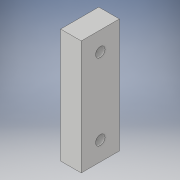
# Autodesk Inventor part: GripperSliderBlock
Saved by Autodesk Inventor 2019 (Build 230136000, 136)
## iProperties
Created: 2019-09-28
Part Number: GripperSliderBlock
Material: Generic
Document SubType Name: Modeling
Designer: james
Density: 1 g/cm^3
Appearance: Default
Mass: 1.5506 g
Surface Area: 10.2449 cm^2
Volume: 1.5506 cm^3
Author: james
Autodesk Inventor part; units mm, degrees
ref_plane "YZ Plane" through (0, 0, 0) normal (1, 0, 0) x (0, 1, 0)
ref_plane "XZ Plane" through (0, 0, 0) normal (0, 1, 0) x (-1, 0, 0)
ref_plane "XY Plane" through (0, 0, 0) normal (0, 0, 1) x (1, 0, 0)
sketch "Sketch1" plane through (0, 0, 0) normal (1, 0, 0) x (0, 1, 0)
  line L0 (12.0622, 21.4347) -> (-26.0378, 21.4347)
  line L1 (-26.0378, 21.4347) -> (-26.0378, 8.7347)
  line L2 (-26.0378, 8.7347) -> (12.0622, 8.7347)
  line L3 (12.0622, 8.7347) -> (12.0622, 21.4347)
  point P0 (0, 0)
  dimension "d0" = 12.7
  dimension "d1" = 38.1
  constraints: 8 end point, 2 parallel, 1 horizontal, 1 perpendicular
  measures "d0" distance of L2.end L0.start
  measures "d1" distance of L0.start L0.end
extrude "Extrusion1" add sketch "Sketch1" along normal blind 6.858
sketch "Sketch2" plane through (6.858, 0, 0) normal (1, 0, 0) x (0, 0, -1)
  line L0 (-8.7347, -26.0378) -> (-8.7347, 12.0622) projected
  line L1 (-8.7347, 12.0622) -> (-21.4347, 12.0622) projected
  point P0 (0, 0)
  point P1 (-15.0847, 5.7122)
  point P2 (-15.0847, -19.6878)
  dimension "d4" = 6.35
  dimension "d5" = 6.35
  dimension "d6" = 31.75
  dimension "d7" = 6.35
  measures "d4" distance from line of L0 point (-15.085, 5.712)
  measures "d5" distance from line of L0 point (-15.085, -19.688)
  measures "d6" distance from line of L1 point (-15.085, -19.688)
  measures "d7" distance from line of L1 point (-15.085, 5.712)
hole "Hole1" at (6.858, 5.7122, 15.0847) at (6.858, -19.6878, 15.0847) direction (-1, 0, 0) diameter 3.175 end through all
body "Solid1"
